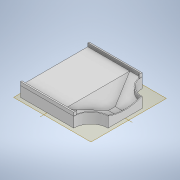
# Autodesk Inventor part: OutputMoneys
Saved by Autodesk Inventor 2020 (Build 240168000, 168)
## iProperties
Created: 2020-03-19
Part Number: OutputMoneys
Material: Типовые
Document SubType Name: Modeling
Designer: CSS38
Density: 1 g/cm^3
Appearance: По умолчанию
Author: CSS38
Autodesk Inventor part; units mm, degrees
ref_plane "YZ Plane" through (0, 0, 0) normal (1, 0, 0) x (0, 1, 0)
ref_plane "XY Plane" through (0, 0, 0) normal (0, 0, 1) x (1, 0, 0)
sketch "Эскиз1" plane through (0, 0, 0) normal (0, 1, 0) x (-1, 0, 0)
  line L0 (77.5, 100) -> (-77.5, 100)
  line L1 (-77.5, 100) -> (-77.5, 50) construction
  line L2 (-77.5, -100) -> (77.5, -100)
  line L3 (77.5, -100) -> (77.5, 100)
  line L4 (77.5, -100) -> (-77.5, 100) construction
  line L5 (-77.5, -100) -> (77.5, 100) construction
  line L6 (-77.5, -50) -> (-127.5, -50) construction
  line L7 (-127.5, -50) -> (-127.5, 0)
  line L8 (-127.5, 50) -> (-77.5, 50) construction
  line L9 (-77.5, 50) -> (-77.5, -50) construction
  line L10 (118.5, 0) -> (-168.5, 0) construction
  line L11 (-127.5, 0) -> (-127.5, 50)
  line L12 (-77.5, -50) -> (-77.5, -100) construction
  line L13 (-77.5, 50) -> (-77.5, -50) construction
  arc A0 (-77.5, -100) -> (-127.5, -50) centre (-127.5, -100) ccw
  arc A1 (-127.5, 50) -> (-77.5, 100) centre (-127.5, 100) ccw
  point P0 (0, 0)
  point P1 (0, 0)
  dimension "d0" = 200
  dimension "d1" = 155
  dimension "d2" = 50
  constraints: 26 end point, 7 parallel, 5 perpendicular, 4 point on circle, 2 centre point, 2 equal length, 2 horizontal, 2 tangent, 1 coincident, 1 midpoint, 1 point on line
  measures "d0" distance of L2.end L0.start
  measures "d1" distance of L2.start L2.end
  measures "d2" distance of L6.start L6.end
extrude "Выдавливание1" add sketch "Эскиз1" along normal blind 3
sketch "Эскиз3" plane through (0, 3, 0) normal (0, 1, 0) x (1, 0, 0)
  arc A0 (77.5, 100) -> (127.5, 50) centre (127.5, 100) ccw projected
  line L0 (127.5, 50) -> (127.5, -50) projected
  arc A1 (127.5, -50) -> (77.5, -100) centre (127.5, -100) ccw projected
  line L1 (77.5, -100) -> (-77.5, -100) projected
  line L2 (-77.5, -100) -> (-77.5, 100) projected
  line L3 (-77.5, 100) -> (77.5, 100) projected
  arc A2 (75.1526, 96) -> (125, 47.5596) centre (127.5, 100) ccw
  line L4 (125, 47.5596) -> (125, -47.5596)
  arc A3 (125, -47.5596) -> (75.1526, -96) centre (127.5, -100) ccw
  line L5 (75.1526, -96) -> (45.1526, -96)
  line L6 (45.1526, 96) -> (75.1526, 96)
  line L7 (45.1526, 96) -> (45.1526, -96)
  dimension "d28" = 2.5
  dimension "d29" = 30
  dimension "d30" = 4
  dimension "d31" = 4
  constraints: 8 end point, 4 point on circle, 2 centre point, 2 perpendicular, 2 other
  measures "d28" distance between parallel lines of L0 L4
  measures "d29" distance of L6.start L6.end
  measures "d30" distance between parallel lines of L3 L6
  measures "d31" distance between parallel lines of L1 L5
extrude "Выдавливание2" add sketch "Эскиз3" along normal blind 27
sketch "Эскиз4" plane through (0, 3, 0) normal (0, 1, 0) x (1, 0, 0)
  line L0 (125, -47.5596) -> (125, 47.5596) projected
  arc A0 (75.1526, 96) -> (125, 47.5596) centre (127.5, 100) ccw projected
  line L1 (75.1526, 96) -> (45.1526, 96) projected
  line L2 (45.1526, 96) -> (45.1526, -96) projected
  line L3 (45.1526, -96) -> (75.1526, -96) projected
  arc A1 (125, -47.5596) -> (75.1526, -96) centre (127.5, -100) ccw projected
  point P0 (0, 0)
extrude "Выдавливание3" add sketch "Эскиз4" along normal up to surface (27 mm away) separate body
sketch "Эскиз5" plane through (45.1526, 3, -96) normal (-1, 0, 0) x (0, 0, 1)
  line L0 (0, 27) -> (86, 2)
  line L1 (86, 2) -> (106, 2)
  line L2 (106, 2) -> (192, 27)
  line L3 (0, 0) -> (192, 0) construction
  line L4 (192, 27) -> (0, 27) projected
  dimension "d32" = 20
  dimension "d33" = 2
  constraints: 6 end point, 1 equal length
  measures "d32" distance of L0.end L1.end
  measures "d33" distance between parallel lines of L3 L1
extrude "Выдавливание4" cut sketch "Эскиз5" against normal through all bodies 2
sketch "Эскиз7" plane through (0, 30, 0) normal (0, 1, 0) x (1, 0, 0)
  line L0 (127.5, -50) -> (127.5, 50) construction
  arc A0 (77.5, 100) -> (127.5, 50) centre (127.5, 100) ccw construction
  line L1 (77.5, 100) -> (-77.5, 100) construction
  line L2 (-77.5, 100) -> (-77.5, -100) construction
  line L3 (-77.5, -100) -> (77.5, -100) construction
  arc A1 (127.5, -50) -> (77.5, -100) centre (127.5, -100) ccw construction
  arc A2 (125, -47.5596) -> (75.1526, -96) centre (127.5, -100) ccw projected
  line L4 (75.1526, -96) -> (45.1526, -96) projected
  line L5 (45.1526, -96) -> (45.1526, 96) projected
  line L6 (45.1526, 96) -> (75.1526, 96) projected
  arc A3 (75.1526, 96) -> (125, 47.5596) centre (127.5, 100) ccw projected
  line L7 (125, 47.5596) -> (125, -47.5596) projected
extrude "Выдавливание5" add sketch "Эскиз7" against normal up to next separate body
sketch "Эскиз8" plane through (75, 30, 0) normal (0, 0, 1) x (1, 0, 0)
  line L0 (-29.8474, 0) -> (0.1526, 0) projected
  line L1 (-29.8474, 0) -> (13.4539, -25)
  line L2 (-29.8474, -25) -> (50, -25) construction
  line L3 (50, -14.0815) -> (50, -25) construction
  line L4 (33.4539, -25) -> (50, -14.0815)
  line L5 (13.4539, -25) -> (33.4539, -25)
  line L6 (0.1526, 0) -> (50, 0) projected
  line L7 (50, 0) -> (50, -14.0815) projected
  point P0 (-75, -30)
  dimension "d34" = 20
  dimension "d35" = 30
  constraints: 6 end point, 2 point on line, 1 collinear
  measures "d34" distance of L4.start L1.end
  measures "d35" angle of L2 L1
extrude "Выдавливание6" cut sketch "Эскиз8" along normal through all both and the other way through all bodies 3
sketch "Эскиз9" plane through (125, 3, -47.5596) normal (-1, 0, 0) x (0, 0, 1)
  line L0 (95.1191, 0) -> (95.1191, 27) construction
  line L1 (0, 27) -> (95.1191, 27) projected
  line L2 (-2.503, 27) -> (0, 27) construction
  line L3 (-2.503, -3) -> (-2.503, 27) construction
  line L4 (97.6221, -3) -> (-2.503, -3) construction
  line L5 (97.6221, 27) -> (97.6221, -3) construction
  line L6 (95.1191, 27) -> (97.6221, 27) construction
  line L7 (0, 0) -> (95.1191, 0) construction
  line L8 (0, 27) -> (0, 0) construction
  line L9 (37.5596, 2) -> (57.5596, 2) construction
  line L10 (57.5596, 2) -> (95.1191, 12.9185) construction
  line L11 (95.1191, 12.9185) -> (95.1191, 0) construction
  line L12 (95.1191, 0) -> (0, 0) construction
  line L13 (0, 0) -> (0, 12.9185) construction
  line L14 (0, 12.9185) -> (37.5596, 2) construction
  line L15 (0, 12.9185) -> (95.1191, 12.9185) construction
  line L16 (95.1191, 12.9185) -> (57.5596, 2) construction
  line L17 (57.5596, 2) -> (37.5596, 2) construction
  line L18 (37.5596, 2) -> (0, 12.9185) construction
  arc A0 (0, 27) -> (95.1191, 27) centre (47.5596, 146.9929) ccw
  point P0 (47.5596, -3)
  dimension "d38" = 5
  constraints: 2 point on circle, 1 centre point
  measures "d38" distance edge to line of A0 L15
extrude "Выдавливание7" cut sketch "Эскиз9" against normal through all bodies 1
sketch "Эскиз10" plane through (0, 30, 0) normal (0, 1, 0) x (1, 0, 0)
  line L0 (77.5, 100) -> (-77.5, 100) projected
  line L1 (-77.5, -100) -> (77.5, -100) projected
  line L2 (-77.5, 100) -> (-77.5, 96)
  line L3 (-77.5, -100) -> (77.5, -100) projected
  arc A0 (75.1526, 96) -> (125, 47.5596) centre (127.5, 100) ccw projected
  line L4 (75.1526, 96) -> (75.1526, 91)
  line L5 (75.1526, 91) -> (77.5, 91)
  arc A1 (77.5, 100) -> (127.5, 50) centre (127.5, 100) ccw projected
  line L6 (77.5, 91) -> (77.5, 100)
  line L7 (75.1526, -96) -> (75.1526, -91)
  line L8 (75.1526, -91) -> (77.5, -91)
  arc A2 (127.5, -50) -> (77.5, -100) centre (127.5, -100) ccw projected
  line L9 (77.5, -91) -> (77.5, -100)
  line L10 (45.1526, 96) -> (75.1526, 96) projected
  line L11 (75.1526, 96) -> (-77.5, 96)
  line L12 (-77.5, -96) -> (75.1526, -96)
  line L13 (-77.5, 96) -> (-77.5, -96) construction
  line L14 (-77.5, -96) -> (-77.5, -100)
  point P0 (0, 0)
  point P1 (75.7772, 91)
  dimension "d43" = 5
  constraints: 22 end point, 10 perpendicular, 2 collinear, 2 tangent, 2 vertical, 1 point on line
  measures "d43" distance of L4.start L4.end
extrude "Выдавливание8" add sketch "Эскиз10" along normal blind 10 separate body contours L6 L5 A0 L10 L11 L2 L0 | L14 L12 L7 L8 L9 L1
